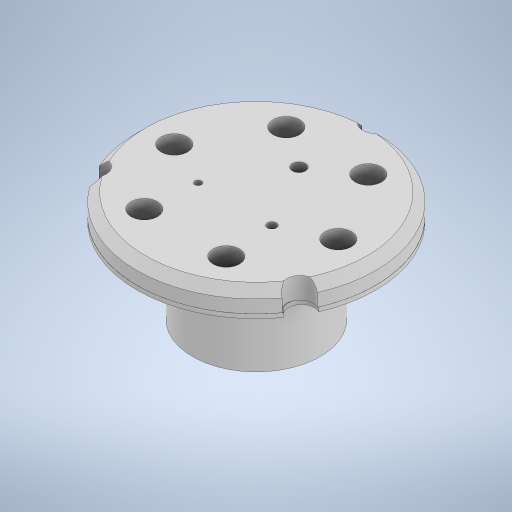
# Autodesk Inventor part: Schneidtrommel
Saved by Autodesk Inventor 2023.2 (Build 272271030, 271C)
## iProperties
Created: 2023-02-11
Part Number: Schneidtrommel
Material: Generic
Document SubType Name: Modeling
Designer: Ayush
Density: 1 g/cm^3
Appearance: Default
Author: Ayush
Autodesk Inventor part; units mm, degrees
ref_plane "YZ Plane" through (0, 0, 0) normal (1, 0, 0) x (0, 1, 0)
ref_plane "XZ Plane" through (0, 0, 0) normal (0, 1, 0) x (-1, 0, 0)
ref_plane "XY Plane" through (0, 0, 0) normal (0, 0, 1) x (1, 0, 0)
sketch "Sketch1" plane through (0, 0, 0) normal (0, 1, 0) x (-1, 0, 0)
  circle A0 centre (0, 0) radius 15
  dimension "d0" = 30
  constraints: 1 centre point, 1 coincident
  measures "d0" diameter of A0
extrude "Extrusion1" add sketch "Sketch1" along normal blind 20
sketch "Sketch2" plane through (0, 20, 0) normal (0, 1, 0) x (1, 0, 0)
  circle A0 centre (0, 0) radius 28
  dimension "d3" = 56
  constraints: 1 centre point, 1 coincident
  measures "d3" diameter of A0
extrude "Extrusion2" add sketch "Sketch2" along normal blind 1
chamfer "Chamfer1" distance 0.01 angle 45 1 edges at (-28, 21, 0) measured on face at (3.0519, 21, 7.6812)
sketch "Sketch3" plane through (0, 21, 0) normal (0, 1, 0) x (1, 0, 0)
  circle A0 centre (-19.2473, 0) radius 3.1
  circle A1 centre (-9.6237, -16.6687) radius 3.1
  circle A2 centre (9.6237, -16.6687) radius 3.1
  circle A3 centre (19.2473, 0) radius 3.1
  circle A4 centre (9.6237, 16.6687) radius 3.1
  circle A5 centre (-9.6237, 16.6687) radius 3.1
  circle A6 centre (0, 0) radius 28 projected
  arc A7 (-3.0455, 27.8339) -> (3.0455, 27.8339) centre (0, 28) ccw
  arc A8 (-22.5821, -16.5544) -> (-25.6276, -11.2795) centre (-24.2487, -14) ccw
  arc A9 (25.6276, -11.2795) -> (22.5821, -16.5544) centre (24.2487, -14) ccw
  circle A10 centre (0, 0) radius 15 projected
  circle A11 centre (0, 10) radius 1.55
  circle A12 centre (8.6603, -5) radius 1.05
  circle A13 centre (-8.6603, -5) radius 0.8
  point P0 (25.6276, -11.2795)
  point P1 (-25.6276, -11.2795)
  dimension "d9" = 6.2
  dimension "d13" = 360
  dimension "d15" = 6.1
  dimension "d18" = 360
  dimension "d21" = 3.1
  dimension "d22" = 2.1
  dimension "d23" = 1.6
  constraints: 12 centre point, 9 point on circle, 1 coincident, 26 other
  measures "d9" diameter of A0
  measures "d15" diameter of A7
  measures "d21" diameter of A11
  measures "d22" diameter of A12
  measures "d23" diameter of A13
extrude "Extrusion3" add sketch "Sketch3" along normal blind 5 contours A6 A9 A8 A7 | A10
sketch "Sketch4" plane through (-9.6237, 21, -16.6687) normal (0, 1, 0) x (1, 0, 0)
  point P0 (9.6237, -16.6687)
  point P1 (-0.0511, -0.0664)
  point P2 (19.3486, -0.121)
  point P3 (29.0211, -16.6244)
  point P4 (19.2295, -33.5187)
  point P5 (0.1688, -33.2971)
  point P6 (-9.5832, -16.7482)
hole "Hole1" at (9.7249, 21, -16.5477) at (19.3974, 21, -0.0443) at (9.6058, 21, 16.85) at (-9.4549, 21, 16.6284) at (-19.2069, 21, 0.0795) at (-9.6748, 21, -16.6023) direction (0, -1, 0) diameter 6.2 end through all
sketch "Sketch5" plane through (8.6603, 21, 5) normal (0, 1, 0) x (1, 0, 0)
  point P0 (-8.6603, 5)
  point P1 (-0.0005, 0.0082)
hole "Hole2" at (8.6598, 21, 4.9918) direction (0, -1, 0) diameter 2.1 end through all
sketch "Sketch6" plane through (0, 21, 0) normal (0, 1, 0) x (1, 0, 0)
  point P0 (0, 0)
  point P1 (-24.3024, -14.1692)
  point P2 (24.3292, -13.7659)
hole "Hole3" at (-24.3024, 21, 14.1692) at (24.3292, 21, 13.7659) direction (0, -1, 0) diameter 6.1 end through all
sketch "Sketch7" plane through (0, 21, 0) normal (0, 1, 0) x (1, 0, 0)
  point P0 (0, 0)
  point P1 (-0.1045, 27.8542)
hole "Hole4" at (-0.1045, 21, -27.8542) direction (0, -1, 0) diameter 6.1 end through all
chamfer "Chamfer2" distance 2 angle 45 3 edges at (0, 26, 28) (24.2487, 26, -14) (-24.2487, 26, -14) measured on face at (-0.1361, 26, 0.2263)
body "Solid1"
